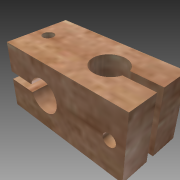
# Autodesk Inventor part: BarClamp_V2
Saved by Autodesk Inventor 2014 (Build 180170000, 170)
## iProperties
Created: 2013-12-17
Part Number: BarClamp_V2
Material: Birch
Document SubType Name: Modeling
Designer: Bram
Density: 0.512 g/cm^3
Appearance: Birch - Natural Medium Gloss
Author: Bram
Autodesk Inventor part; units mm, degrees
ref_plane "YZ Plane" through (0, 0, 0) normal (1, 0, 0) x (0, 1, 0)
ref_plane "XZ Plane" through (0, 0, 0) normal (0, 1, 0) x (-1, 0, 0)
ref_plane "XY Plane" through (0, 0, 0) normal (0, 0, 1) x (1, 0, 0)
sketch "Sketch1" plane through (0, 0, 0) normal (1, 0, 0) x (0, 1, 0)
  line L0 (0, 0) -> (16, 0)
  line L1 (16, 0) -> (16, 16)
  line L2 (16, 16) -> (0, 16)
  line L3 (0, 16) -> (0, 0)
  dimension "d0" = 16
  dimension "d1" = 16
  constraints: 8 end point, 2 parallel, 1 horizontal, 1 perpendicular
  measures "d0" distance of L2.end L1.end
  measures "d1" distance of L1.end L0.end
extrude "Extrusion1" add sketch "Sketch1" along normal blind 32
sketch "Sketch2" plane through (0, 0, 16) normal (0, 0, 1) x (1, 0, 0)
  line L0 (32, 16) -> (32, 0) projected
  circle A0 centre (21, 8) radius 4
  line L1 (32, 8) -> (32, 9)
  line L2 (32, 9) -> (32, 7)
  line L3 (32, 7) -> (24.873, 7)
  line L4 (32, 9) -> (24.873, 9)
  circle A1 centre (3.5, 8) radius 1.5
  dimension "d5" = 8
  dimension "d6" = 1
  dimension "d7" = 2
  dimension "d9" = 3
  constraints: 8 end point, 2 centre point, 2 point on circle, 2 point on line, 1 midpoint, 1 perpendicular
  measures "d5" diameter of A0
  measures "d6" distance of L1.start L1.end
  measures "d7" distance of L1.end L2.end
  measures "d9" diameter of A1
extrude "Extrusion2" cut sketch "Sketch2" against normal blind 32
sketch "Sketch3" plane through (0, 16, 16) normal (0, 1, 0) x (1, 0, 0)
  line L0 (0, 16) -> (0, 0) projected
  line L1 (0, 0) -> (32, 0) projected
  line L2 (32, 16) -> (32, 0) projected
  line L3 (0, 16) -> (32, 16) projected
  line L4 (16, 16) -> (16, 0)
  line L5 (16, 8) -> (11, 8)
  circle A0 centre (11, 8) radius 4
  line L6 (0, 8) -> (0, 9)
  line L7 (0, 9) -> (7.127, 9)
  line L8 (0, 8) -> (0, 7)
  line L9 (0, 7) -> (7.127, 7)
  line L10 (32, 8) -> (28.5, 8)
  circle A1 centre (28.5, 8) radius 1.5
  dimension "d12" = 5
  dimension "d13" = 8
  dimension "d14" = 1
  dimension "d15" = 1
  dimension "d16" = 3.5
  dimension "d17" = 3
  constraints: 14 end point, 5 midpoint, 3 perpendicular, 2 centre point, 2 coincident, 2 point on circle, 2 point on line, 1 parallel
  measures "d12" distance of L5.start L5.end
  measures "d13" diameter of A0
  measures "d14" distance of L6.start L6.end
  measures "d15" distance of L6.start L8.end
  measures "d16" distance of L10.start L10.end
  measures "d17" diameter of A1
extrude "Extrusion3" cut sketch "Sketch3" against normal blind 32 contours L7 A0 L9 L0 | A1 | A0
body "Solid1"
